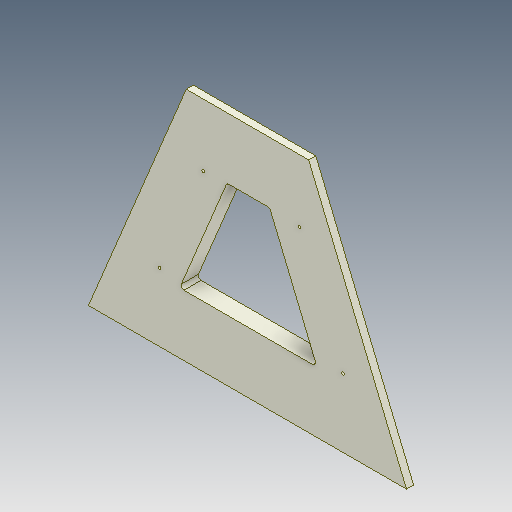
# Autodesk Inventor part: Stage2
Saved by Autodesk Inventor 2018.2 (Build 222227000, 227)
## iProperties
Created: 2018-11-01
Part Number: Stage2
Material: ABS-Kunststoff
Document SubType Name: Modeling
Designer: M.Knabel
Density: 1.06 g/cm^3
Appearance: Glatt - Elfenbein
Mass: 26.953 g
Surface Area: 131.178 cm^2
Volume: 25.4274 cm^3
Author: M.Knabel
Autodesk Inventor part; units mm, degrees
ref_plane "YZ Plane" through (0, 0, 0) normal (1, 0, 0) x (0, 1, 0)
ref_plane "XZ Plane" through (0, 0, 0) normal (0, 1, 0) x (-1, 0, 0)
ref_plane "XY Plane" through (0, 0, 0) normal (0, 0, 1) x (1, 0, 0)
sketch "Skizze1" plane through (0, 0, 0) normal (0, 1, 0) x (-1, 0, 0)
  line L0 (-21.5, 41.5) -> (21.5, 41.5)
  line L1 (21.5, 41.5) -> (55.8797, -41.5)
  line L2 (55.8797, -41.5) -> (-55.8797, -41.5)
  line L3 (-55.8797, -41.5) -> (-21.5, 41.5)
  line L4 (78.2316, 0) -> (-78.2316, 0) construction
  line L5 (0, -58.1) -> (0, 58.1) construction
  point P0 (0, 0)
  dimension "d0" = 83
  dimension "d1" = 112.5
  dimension "d2" = 43
  constraints: 8 end point, 1 horizontal, 1 parallel, 2 other
  measures "d0" distance between parallel lines of L2 L0
  measures "d1" angle of L0 L3
  measures "d2" distance of L0.start L0.end
extrude "Extrusion1" add sketch "Skizze1" along normal blind 6
sketch "Skizze2" plane through (0, 6, 0) normal (0, 1, 0) x (1, 0, 0)
  line L0 (-21.5, -41.5) -> (21.5, -41.5) projected
  line L1 (21.5, -41.5) -> (55.8797, 41.5) projected
  line L2 (55.8797, 41.5) -> (-55.8797, 41.5) projected
  line L3 (-55.8797, 41.5) -> (-21.5, -41.5) projected
  line L4 (-48.3967, 36.5) -> (48.3967, 36.5)
  line L5 (48.3967, 36.5) -> (18.1591, -36.5)
  line L6 (18.1591, -36.5) -> (-18.1591, -36.5)
  line L7 (-18.1591, -36.5) -> (-48.3967, 36.5)
  point P0 (0, 0)
  dimension "d5" = 5
  constraints: 8 end point, 3 other
  measures "d5" distance between parallel lines of L2 L4
extrude "Extrusion2" cut sketch "Skizze2" against normal blind 3.5
sketch "Skizze3" plane through (0, 6, 0) normal (0, 1, 0) x (1, 0, 0)
  circle A0 centre (33.5685, 17.5) radius 4 projected
  circle A1 centre (18.2426, -19.5) radius 4 projected
  line L0 (63.0664, 44.5) -> (12.5288, 44.5) projected
  arc A2 (12.5288, 44.5) -> (-9.8319, 44.5) centre (1.3485, 34.5) ccw projected
  line L1 (-9.8319, 44.5) -> (-60.3695, 44.5) projected
  line L2 (-60.3695, 44.5) -> (-23.5045, -44.5) projected
  line L3 (-23.5045, -44.5) -> (26.2015, -44.5) projected
  line L4 (26.2015, -44.5) -> (63.0664, 44.5) projected
  circle A3 centre (-15.5457, -19.5) radius 4 projected
  circle A4 centre (-30.8716, 17.5) radius 4 projected
  point P0 (0, 0)
hole "Bohrung1" at (-30.8716, 6, -17.5) at (33.5685, 6, -17.5) at (18.2426, 6, 19.5) at (-15.5457, 6, 19.5) direction (0, -1, 0) diameter 1 end through all
sketch "Skizze4" plane through (0, 6, 0) normal (0, 1, 0) x (1, 0, 0)
  line L0 (58.5766, 41.5) -> (-55.8797, 41.5) construction
  line L1 (-55.8797, 41.5) -> (-21.5, -41.5) construction
  line L2 (-21.5, -41.5) -> (24.1969, -41.5) construction
  line L3 (55.8797, 41.5) -> (21.5, -41.5) construction
  line L4 (22.4292, -40.7678) -> (56.8089, 42.2322) construction
  line L5 (-23.8211, 20.0791) -> (24.4471, 20.0791)
  line L6 (24.4471, 20.0791) -> (7.813, -20.0791)
  line L7 (7.813, -20.0791) -> (-7.187, -20.0791)
  line L8 (-7.187, -20.0791) -> (-23.8211, 20.0791)
  point P0 (0, 0)
  dimension "d15" = 15
  constraints: 8 end point, 3 other
  measures "d15" distance of L6.end L7.end
extrude "Extrusion3" cut sketch "Skizze4" against normal through all
fillet "Rundung1" radius 1 4 edges at (24.4471, 3, -20.0791) (7.813, 3, 20.0791) (-7.187, 3, 20.0791) (-23.8211, 3, -20.0791)
